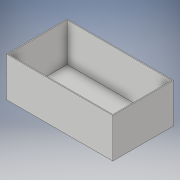
# Autodesk Inventor part: containerofm2
Saved by Autodesk Inventor 2019 (Build 230136000, 136)
## iProperties
Created: 2020-03-04
Part Number: containerofm2
Material: Generic
Document SubType Name: Modeling
Designer: Lenovo
Density: 1 g/cm^3
Appearance: Default
Author: Lenovo
Autodesk Inventor part; units mm, degrees
ref_plane "YZ Plane" through (0, 0, 0) normal (1, 0, 0) x (0, 1, 0)
ref_plane "XZ Plane" through (0, 0, 0) normal (0, 1, 0) x (-1, 0, 0)
ref_plane "XY Plane" through (0, 0, 0) normal (0, 0, 1) x (1, 0, 0)
sketch "Sketch1" plane through (0, 0, 0) normal (0, 1, 0) x (-1, 0, 0)
  line L0 (0, 0) -> (350, 0)
  line L1 (350, 0) -> (350, 200)
  line L2 (350, 200) -> (0, 200)
  line L3 (0, 200) -> (0, 0)
  dimension "d0" = 350
  dimension "d1" = 200
  constraints: 8 end point, 2 parallel, 1 horizontal, 1 perpendicular
  measures "d0" distance of L2.end L1.end
  measures "d1" distance of L1.end L0.end
extrude "Extrusion1" add sketch "Sketch1" along normal blind 130
sketch "Sketch2" plane through (0, 130, 0) normal (0, 1, 0) x (1, 0, 0)
  line L0 (0, 0) -> (0, -3)
  line L1 (0, -3) -> (-3, -3)
  line L2 (-3, -3) -> (-347, -3)
  line L3 (-347, -3) -> (-347, -197)
  line L4 (-347, -197) -> (-3, -197)
  line L5 (-3, -197) -> (-3, -3)
  dimension "d4" = 3
  dimension "d5" = 3
  dimension "d6" = 344
  dimension "d7" = 194
  constraints: 12 end point, 2 parallel, 2 perpendicular, 1 horizontal, 1 vertical
  measures "d4" distance of L0.start L0.end
  measures "d5" distance of L0.end L1.end
  measures "d6" distance of L4.end L3.end
  measures "d7" distance of L3.end L2.end
extrude "Extrusion2" cut sketch "Sketch2" against normal blind 127
body "Solid1"
